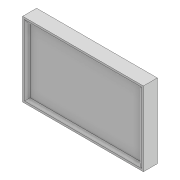
# Autodesk Inventor part: Display_Dummy
Saved by Autodesk Inventor 2020 (Build 240168000, 168)
## iProperties
Created: 2022-01-25
Part Number: Display_Dummy
Material: Generisch
Document SubType Name: Modeling
Designer: Julian Uhl
Density: 1 g/cm^3
Appearance: Vorgabe
Author: Julian Uhl
Autodesk Inventor part; units mm, degrees
ref_plane "YZ Plane" through (0, 0, 0) normal (1, 0, 0) x (0, 1, 0)
ref_plane "XZ Plane" through (0, 0, 0) normal (0, 1, 0) x (-1, 0, 0)
ref_plane "XY Plane" through (0, 0, 0) normal (0, 0, 1) x (1, 0, 0)
sketch "Skizze2" plane through (0, 0, 0) normal (0, 0, 1) x (1, 0, 0)
  line L0 (-26, 0) -> (156, 0) projected
  line L1 (0, -16) -> (0, 96) projected
  line L2 (0, 0) -> (130, 0)
  line L3 (130, 0) -> (130, 80)
  line L4 (130, 80) -> (0, 80)
  line L5 (0, 80) -> (0, 0)
  point P0 (0, 80)
  dimension "d0" = 80
  dimension "d1" = 130
  constraints: 8 end point, 2 parallel, 1 horizontal, 1 perpendicular
  measures "d0" distance between parallel lines of L0 L4
  measures "d1" distance between parallel lines of L3 L5
extrude "Extrusion1" add sketch "Skizze2" along normal blind 15
sketch "Skizze3" plane through (0, 0, 15) normal (0, 0, 1) x (1, 0, 0)
  line L0 (5, 75) -> (125, 75)
  line L1 (125, 75) -> (125, 5)
  line L2 (125, 5) -> (5, 5)
  line L3 (5, 5) -> (5, 75)
  line L4 (130, 80) -> (0, 80) projected
  line L5 (130, 0) -> (130, 80) projected
  line L6 (0, 0) -> (130, 0) projected
  line L7 (0, 80) -> (0, 0) projected
  dimension "d4" = 5
  dimension "d5" = 5
  dimension "d6" = 5
  dimension "d7" = 5
  constraints: 8 end point, 2 parallel, 1 horizontal, 1 perpendicular
  measures "d4" distance between parallel lines of L0 L4
  measures "d5" distance between parallel lines of L5 L1
  measures "d6" distance between parallel lines of L6 L2
  measures "d7" distance between parallel lines of L7 L3
extrude "Extrusion2" cut sketch "Skizze3" against normal blind 3 contours L0 L1 L2 L3
fillet "Rundung1" radius 3 4 edges at (65, 75, 15) (5, 40, 15) (65, 5, 15) (125, 40, 15)
